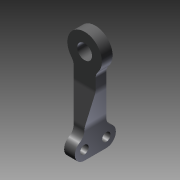
# Autodesk Inventor part: 205-S-SA
Saved by Autodesk Inventor 2011 SP1 (Build 150282100, 282)
## iProperties
Created: 2017-03-01
Part Number: 205-S-SA
Catalog Web Link: www.cadenas.de
Description: S-SA-SU-S-Spannarm
Vendor: DESTACO
Document SubType Name: Modeling
Designer: psAdmin
Manufacturer: DESTACO
Mass: 0.682974 g
Surface Area: 7.68733 cm^2
Volume: 0.682974 cm^3
Density: 1 g/cm^3
Category: PARTsolutions
Company: DESTACO
Title: 205-S-SA
Author: Cadenas PARTsolutions
Comments: S-Spannarm
PSOL_IDENT_0: {$CADENAS_DATA\23d-libs\destaco\destaco_gmbh\man_spann\horizontalspanner\standard\su_parts\s_spannar
PSOL_IDENT_1: m_su.prj},161 {VTYP=3D},{NB=205-S-SA},{LINA=205-S-SA},{NN=S-SA-SU},{DATE=20.09.2016 07:53:12},{GEOMD
PSOL_IDENT_2: ATE=01.12.2015 13:22:00},{VERSION=v1},{LINEID=20},{LINESUBID=-1},{WBVAR=}  {NB=205-S-SA},{LINA=205-S
PSOL_IDENT_3: -SA},{KT=DUMMY},{MODELL=205-S-SA},{SIZE=1},{MOD=1.000}
NN: S-SA-SU
NT: S-Spannarm
NB: 205-S-SA
NBSYN: $MODELL.
LINA: 205-S-SA
MODELL: 205-S-SA
SIZE: 1
MOD: 1.000
SUPPLIER: DESTACO
ARTICLENO: 205-S-SA
BOMINFO: 205-S-SA
CREATOR: CADENAS GmbH
Autodesk Inventor part; units mm, degrees
sketch "Skizze_1" plane through (0, 0, 0) normal (1, 0, 0) x (0, 1, 0)
  line L0 (4.724, 30) -> (1.626, 30)
  line L1 (1.626, 30) -> (1.626, 14.9265)
  arc A0 (1.5502, 14.0803) -> (1.626, 14.9265) centre (-3.134, 14.9265) ccw
  line L2 (1.5502, 14.0803) -> (0.0758, 5.9197)
  arc A1 (0.0758, 5.9197) -> (0, 5.0735) centre (4.76, 5.0735) ccw
  line L3 (0, 5.0735) -> (0, 4.8116)
  arc A2 (-1.389, 2.4058) -> (0, 4.8116) centre (-2.778, 4.8116) ccw
  arc A3 (-1.389, 2.4058) -> (0, -2.778) centre (0, 0) ccw
  line L4 (0, -2.778) -> (6.35, -2.778)
  arc A4 (6.35, -2.778) -> (7.739, 2.4058) centre (6.35, 0) ccw
  arc A5 (6.35, 4.8116) -> (7.739, 2.4058) centre (9.128, 4.8116) ccw
  line L5 (6.35, 4.8116) -> (6.35, 5.0735)
  arc A6 (6.35, 5.0735) -> (6.2742, 5.9197) centre (1.59, 5.0735) ccw
  line L6 (6.2742, 5.9197) -> (4.7998, 14.0803)
  arc A7 (4.724, 14.9265) -> (4.7998, 14.0803) centre (9.484, 14.9265) ccw
  line L7 (4.724, 14.9265) -> (4.724, 30)
  constraints: 16 end point, 16 point on circle, 8 centre point
extrude "Extrusion1" add sketch "Skizze_1" along normal mid plane 10
sketch "Skizze_2" plane through (0, 0, 0) normal (0, 1, 0) x (-1, 0, 0)
  line L0 (39, 78) -> (-69, 78)
  line L1 (-69, 78) -> (-69, -55)
  line L2 (-69, -55) -> (39, -55)
  line L3 (39, -55) -> (39, 78)
  arc A0 (3.8268, 19.769) -> (0, 27.987) centre (0, 22.987) ccw
  arc A1 (0, 27.987) -> (-3.8268, 19.769) centre (0, 22.987) ccw
  arc A2 (-3.175, 17.9811) -> (-3.8268, 19.769) centre (-5.953, 17.9811) ccw
  line L4 (-3.175, 17.9811) -> (-3.175, 15.2476)
  arc A3 (-3.175, 15.2476) -> (-3.0253, 13.5657) centre (6.35, 15.2476) ccw
  line L5 (-3.0253, 13.5657) -> (-1.6987, 6.1703)
  arc A4 (-1.549, 4.4884) -> (-1.6987, 6.1703) centre (-11.074, 4.4884) ccw
  line L6 (-1.549, 4.4884) -> (-1.549, -2.788)
  line L7 (-1.549, -2.788) -> (1.549, -2.788)
  line L8 (1.549, -2.788) -> (1.549, 4.4884)
  arc A5 (1.6987, 6.1703) -> (1.549, 4.4884) centre (11.074, 4.4884) ccw
  line L9 (1.6987, 6.1703) -> (3.0253, 13.5657)
  arc A6 (3.0253, 13.5657) -> (3.175, 15.2476) centre (-6.35, 15.2476) ccw
  line L10 (3.175, 15.2476) -> (3.175, 17.9811)
  arc A7 (3.8268, 19.769) -> (3.175, 17.9811) centre (5.953, 17.9811) ccw
  constraints: 22 end point, 16 point on circle, 8 centre point
extrude "Extrusion2" cut sketch "Skizze_2" along normal mid plane 40
sketch "Skizze_3" plane through (0, 0, 0) normal (1, 0, 0) x (0, 1, 0)
  line L0 (10, 22.987) -> (-10, 22.987)
  line L1 (-10, 22.987) -> (-10, 25.137)
  line L2 (-10, 25.137) -> (10, 25.137)
  line L3 (10, 25.137) -> (10, 22.987)
  line L4 (10, 22.987) -> (-10, 22.987)
  constraints: 10 end point
revolve "Revolution1" cut sketch "Skizze_3" angle 360 about axis through (0, 10, 22.987) along (0, 1, 0)
sketch "Skizze_4" plane through (0, 0, 0) normal (0, 0, 1) x (1, 0, 0)
  line L0 (10, 0) -> (-10, 0)
  line L1 (-10, 0) -> (-10, 1.219)
  line L2 (-10, 1.219) -> (10, 1.219)
  line L3 (10, 1.219) -> (10, 0)
  line L4 (10, 0) -> (-10, 0)
  constraints: 10 end point
revolve "Revolution2" cut sketch "Skizze_4" angle 360 about axis through (10, 0, 0) along (1, 0, 0)
sketch "Skizze_5" plane through (0, 0, 0) normal (0, 0, 1) x (1, 0, 0)
  line L0 (10, 6.35) -> (-10, 6.35)
  line L1 (-10, 6.35) -> (-10, 7.569)
  line L2 (-10, 7.569) -> (10, 7.569)
  line L3 (10, 7.569) -> (10, 6.35)
  line L4 (10, 6.35) -> (-10, 6.35)
  constraints: 10 end point
revolve "Revolution3" cut sketch "Skizze_5" angle 360 about axis through (10, 6.35, 0) along (1, 0, 0)
ref_plane "SA1_XY" through (0, 0, 0) normal (1, 0, 0) x (0, 0, -1)
ref_plane "SA1_YZ" through (0, 0, 0) normal (0, 0, -1) x (0, 1, 0)
ref_plane "SA1_ZX" through (0, 0, 0) normal (0, 1, 0) x (1, 0, 0)
ref_plane "SA2_XY" through (0, 6.35, 0) normal (1, 0, 0) x (0, 0, -1)
ref_plane "SA2_YZ" through (0, 6.35, 0) normal (0, 0, -1) x (0, 1, 0)
ref_plane "SA2_ZX" through (0, 6.35, 0) normal (0, 1, 0) x (1, 0, 0)
ref_plane "SA3_XY" through (0, 3.175, 22.987) normal (0, 1, 0) x (1, 0, 0)
ref_plane "SA3_YZ" through (0, 3.175, 22.987) normal (1, 0, 0) x (0, 0, -1)
ref_plane "SA3_ZX" through (0, 3.175, 22.987) normal (0, 0, -1) x (0, 1, 0)
ref_plane "b_left_XY" through (0, 1.626, 27.987) normal (1, 0, 0) x (0, 0, -1)
ref_plane "b_left_YZ" through (0, 1.626, 27.987) normal (0, 0, -1) x (0, 1, 0)
ref_plane "b_left_ZX" through (0, 1.626, 27.987) normal (0, 1, 0) x (1, 0, 0)
ref_plane "r_top_XY" through (0, 9.128, 0) normal (1, 0, 0) x (0, 0, -1)
ref_plane "r_top_YZ" through (0, 9.128, 0) normal (0, 0, -1) x (0, 1, 0)
ref_plane "r_top_ZX" through (0, 9.128, 0) normal (0, 1, 0) x (1, 0, 0)
ref_plane "z_left_XY" through (0, 4.724, 27.987) normal (1, 0, 0) x (0, 0, -1)
ref_plane "z_left_YZ" through (0, 4.724, 27.987) normal (0, 0, -1) x (0, 1, 0)
ref_plane "z_left_ZX" through (0, 4.724, 27.987) normal (0, 1, 0) x (1, 0, 0)
body "Solid1"
